Autodesk Inventor part; units mm, degrees
(part 3 of 3)
  line L539 (30.1684, 3.8123) -> (30.5948, 3.6909)
  line L540 (30.5948, 3.6909) -> (31.0222, 3.5524)
  line L541 (31.0222, 3.5524) -> (31.0829, 2.9751)
  line L542 (31.0829, 2.9751) -> (30.6936, 2.7507)
  line L543 (30.6936, 2.7507) -> (30.3018, 2.5433)
  line L544 (30.3018, 2.5433) -> (29.9075, 2.3538)
  line L545 (29.9075, 2.3538) -> (29.511, 2.1835)
  line L546 (29.511, 2.1835) -> (29.1124, 2.0344)
  line L547 (29.1124, 2.0344) -> (28.9123, 1.9688)
  line L548 (28.9123, 1.9688) -> (28.812, 1.9385)
  line L549 (28.812, 1.9385) -> (28.7116, 1.9099)
  line L550 (28.7116, 1.9099) -> (28.754, 1.1017)
  line L551 (28.754, 1.1017) -> (28.8568, 1.0838)
  line L552 (28.8568, 1.0838) -> (28.9597, 1.0641)
  line L553 (28.9597, 1.0641) -> (29.1656, 1.0198)
  line L554 (29.1656, 1.0198) -> (29.5776, 0.9132)
  line L555 (29.5776, 0.9132) -> (29.9897, 0.7853)
  line L556 (29.9897, 0.7853) -> (30.4016, 0.638)
  line L557 (30.4016, 0.638) -> (30.813, 0.4727)
  line L558 (30.813, 0.4727) -> (31.2236, 0.2903)
  line L559 (31.2236, 0.2903) -> (31.2236, -0.2903)
  line L560 (31.2236, -0.2903) -> (30.813, -0.4727)
  line L561 (30.813, -0.4727) -> (30.4016, -0.638)
  line L562 (30.4016, -0.638) -> (29.9897, -0.7853)
  line L563 (29.9897, -0.7853) -> (29.5776, -0.9132)
  line L564 (29.5776, -0.9132) -> (29.1656, -1.0198)
  line L565 (29.1656, -1.0198) -> (28.9597, -1.0641)
  line L566 (28.9597, -1.0641) -> (28.8568, -1.0838)
  line L567 (28.8568, -1.0838) -> (28.754, -1.1017)
  line L568 (28.754, -1.1017) -> (28.7116, -1.9099)
  line L569 (28.7116, -1.9099) -> (28.812, -1.9385)
  line L570 (28.812, -1.9385) -> (28.9123, -1.9688)
  line L571 (28.9123, -1.9688) -> (29.1124, -2.0344)
  line L572 (29.1124, -2.0344) -> (29.511, -2.1835)
  line L573 (29.511, -2.1835) -> (29.9075, -2.3538)
  line L574 (29.9075, -2.3538) -> (30.3018, -2.5433)
  line L575 (30.3018, -2.5433) -> (30.6936, -2.7507)
  line L576 (30.6936, -2.7507) -> (31.0829, -2.9751)
  line L577 (31.0829, -2.9751) -> (31.0222, -3.5524)
  line L578 (31.0222, -3.5524) -> (30.5948, -3.6909)
  line L579 (30.5948, -3.6909) -> (30.1684, -3.8124)
  line L580 (30.1684, -3.8124) -> (29.7433, -3.9158)
  line L581 (29.7433, -3.9158) -> (29.3201, -3.9999)
  line L582 (29.3201, -3.9999) -> (28.8992, -4.0628)
  line L583 (28.8992, -4.0628) -> (28.6898, -4.0854)
  line L584 (28.6898, -4.0854) -> (28.5855, -4.0942)
  line L585 (28.5855, -4.0942) -> (28.4813, -4.1013)
  line L586 (28.4813, -4.1013) -> (28.3547, -4.9006)
  line L587 (28.3547, -4.9006) -> (28.4516, -4.9395)
  line L588 (28.4516, -4.9395) -> (28.5481, -4.9802)
  line L589 (28.5481, -4.9802) -> (28.7403, -5.0663)
  line L590 (28.7403, -5.0663) -> (29.1211, -5.2563)
  line L591 (29.1211, -5.2563) -> (29.4976, -5.4671)
  line L592 (29.4976, -5.4671) -> (29.8699, -5.6968)
  line L593 (29.8699, -5.6968) -> (30.2379, -5.944)
  line L594 (30.2379, -5.944) -> (30.6016, -6.2078)
  line L595 (30.6016, -6.2078) -> (30.4809, -6.7757)
  line L596 (30.4809, -6.7757) -> (30.0414, -6.8687)
  line L597 (30.0414, -6.8687) -> (29.6046, -6.9449)
  line L598 (29.6046, -6.9449) -> (29.1711, -7.0034)
  line L599 (29.1711, -7.0034) -> (28.7414, -7.0428)
  line L600 (28.7414, -7.0428) -> (28.3162, -7.0614)
  line L601 (28.3162, -7.0614) -> (28.1056, -7.0619)
  line L602 (28.1056, -7.0619) -> (28.0009, -7.0598)
  line L603 (28.0009, -7.0598) -> (27.8966, -7.0559)
  line L604 (27.8966, -7.0559) -> (27.6871, -7.8377)
  line L605 (27.6871, -7.8377) -> (27.7794, -7.8865)
  line L606 (27.7794, -7.8865) -> (27.8711, -7.937)
  line L607 (27.8711, -7.937) -> (28.0532, -8.0428)
  line L608 (28.0532, -8.0428) -> (28.4122, -8.2714)
  line L609 (28.4122, -8.2714) -> (28.7646, -8.5205)
  line L610 (28.7646, -8.5205) -> (29.1108, -8.7878)
  line L611 (29.1108, -8.7878) -> (29.451, -9.0722)
  line L612 (29.451, -9.0722) -> (29.7851, -9.3725)
  line L613 (29.7851, -9.3725) -> (29.6057, -9.9247)
  line L614 (29.6057, -9.9247) -> (29.1588, -9.9713)
  line L615 (29.1588, -9.9713) -> (28.7165, -10.0014)
  line L616 (28.7165, -10.0014) -> (28.2792, -10.0142)
  line L617 (28.2792, -10.0142) -> (27.8478, -10.0085)
  line L618 (27.8478, -10.0085) -> (27.423, -9.9825)
  line L619 (27.423, -9.9825) -> (27.2135, -9.9611)
  line L620 (27.2135, -9.9611) -> (27.1095, -9.948)
  line L621 (27.1095, -9.948) -> (27.0062, -9.9333)
  line L622 (27.0062, -9.9333) -> (26.7162, -10.6888)
  line L623 (26.7162, -10.6888) -> (26.8028, -10.747)
  line L624 (26.8028, -10.747) -> (26.8888, -10.8068)
  line L625 (26.8888, -10.8068) -> (27.0589, -10.9311)
  line L626 (27.0589, -10.9311) -> (27.3919, -11.196)
  line L627 (27.3919, -11.196) -> (27.7164, -11.4805)
  line L628 (27.7164, -11.4805) -> (28.0328, -11.7826)
  line L629 (28.0328, -11.7826) -> (28.3413, -12.1009)
  line L630 (28.3413, -12.1009) -> (28.6422, -12.4346)
  line L631 (28.6422, -12.4346) -> (28.4061, -12.965)
  line L632 (28.4061, -12.965) -> (27.9568, -12.9646)
  line L633 (27.9568, -12.9646) -> (27.5137, -12.9483)
  line L634 (27.5137, -12.9483) -> (27.0776, -12.9153)
  line L635 (27.0776, -12.9153) -> (26.649, -12.8646)
  line L636 (26.649, -12.8646) -> (26.2293, -12.7943)
  line L637 (26.2293, -12.7943) -> (26.0232, -12.7511)
  line L638 (26.0232, -12.7511) -> (25.9212, -12.7272)
  line L639 (25.9212, -12.7272) -> (25.82, -12.7018)
  line L640 (25.82, -12.7018) -> (25.4526, -13.4229)
  line L641 (25.4526, -13.4229) -> (25.5327, -13.4898)
  line L642 (25.5327, -13.4898) -> (25.6119, -13.5583)
  line L643 (25.6119, -13.5583) -> (25.768, -13.6996)
  line L644 (25.768, -13.6996) -> (26.0716, -13.9979)
  line L645 (26.0716, -13.9979) -> (26.3645, -14.3148)
  line L646 (26.3645, -14.3148) -> (26.6476, -14.6483)
  line L647 (26.6476, -14.6483) -> (26.9212, -14.9971)
  line L648 (26.9212, -14.9971) -> (27.1855, -15.3604)
  line L649 (27.1855, -15.3604) -> (26.8952, -15.8632)
  line L650 (26.8952, -15.8632) -> (26.4485, -15.8158)
  line L651 (26.4485, -15.8158) -> (26.0096, -15.7533)
  line L652 (26.0096, -15.7533) -> (25.5792, -15.675)
  line L653 (25.5792, -15.675) -> (25.1583, -15.5797)
  line L654 (25.1583, -15.5797) -> (24.7482, -15.466)
  line L655 (24.7482, -15.466) -> (24.5478, -15.4014)
  line L656 (24.5478, -15.4014) -> (24.4488, -15.367)
  line L657 (24.4488, -15.367) -> (24.3508, -15.3311)
  line L658 (24.3508, -15.3311) -> (23.91, -16.0099)
  line L659 (23.91, -16.0099) -> (23.9827, -16.0848)
  line L660 (23.9827, -16.0848) -> (24.0544, -16.1612)
  line L661 (24.0544, -16.1612) -> (24.1949, -16.3181)
  line L662 (24.1949, -16.3181) -> (24.4656, -16.6465)
  line L663 (24.4656, -16.6465) -> (24.7238, -16.9922)
  line L664 (24.7238, -16.9922) -> (24.9704, -17.3534)
  line L665 (24.9704, -17.3534) -> (25.2061, -17.729)
  line L666 (25.2061, -17.729) -> (25.431, -18.1179)
  line L667 (25.431, -18.1179) -> (25.0898, -18.5876)
  line L668 (25.0898, -18.5876) -> (24.6504, -18.4938)
  line L669 (24.6504, -18.4938) -> (24.2204, -18.3858)
  line L670 (24.2204, -18.3858) -> (23.8006, -18.2628)
  line L671 (23.8006, -18.2628) -> (23.392, -18.1241)
  line L672 (23.392, -18.1241) -> (22.996, -17.9681)
  line L673 (22.996, -17.9681) -> (22.8034, -17.883)
  line L674 (22.8034, -17.883) -> (22.7086, -17.8384)
  line L675 (22.7086, -17.8384) -> (22.6149, -17.7925)
  line L676 (22.6149, -17.7925) -> (22.1056, -18.4214)
  line L677 (22.1056, -18.4214) -> (22.17, -18.5035)
  line L678 (22.17, -18.5035) -> (22.2333, -18.587)
  line L679 (22.2333, -18.587) -> (22.3566, -18.7577)
  line L680 (22.3566, -18.7577) -> (22.5915, -19.1126)
  line L681 (22.5915, -19.1126) -> (22.8122, -19.4834)
  line L682 (22.8122, -19.4834) -> (23.0197, -19.8685)
  line L683 (23.0197, -19.8685) -> (23.2148, -20.2666)
  line L684 (23.2148, -20.2666) -> (23.3979, -20.6769)
  line L685 (23.3979, -20.6769) -> (23.0094, -21.1084)
  line L686 (23.0094, -21.1084) -> (22.5822, -20.9692)
  line L687 (22.5822, -20.9692) -> (22.1659, -20.8168)
  line L688 (22.1659, -20.8168) -> (21.7612, -20.6506)
  line L689 (21.7612, -20.6506) -> (21.3694, -20.4699)
  line L690 (21.3694, -20.4699) -> (20.9919, -20.2734)
  line L691 (20.9919, -20.2734) -> (20.8092, -20.1686)
  line L692 (20.8092, -20.1686) -> (20.7196, -20.1144)
  line L693 (20.7196, -20.1144) -> (20.6312, -20.0589)
  line L694 (20.6312, -20.0589) -> (20.0589, -20.6312)
  line L695 (20.0589, -20.6312) -> (20.1144, -20.7196)
  line L696 (20.1144, -20.7196) -> (20.1686, -20.8092)
  line L697 (20.1686, -20.8092) -> (20.2734, -20.9919)
  line L698 (20.2734, -20.9919) -> (20.4699, -21.3694)
  line L699 (20.4699, -21.3694) -> (20.6506, -21.7612)
  line L700 (20.6506, -21.7612) -> (20.8168, -22.1659)
  line L701 (20.8168, -22.1659) -> (20.9692, -22.5822)
  line L702 (20.9692, -22.5822) -> (21.1084, -23.0094)
  line L703 (21.1084, -23.0094) -> (20.6769, -23.3979)
  line L704 (20.6769, -23.3979) -> (20.2666, -23.2148)
  line L705 (20.2666, -23.2148) -> (19.8685, -23.0197)
  line L706 (19.8685, -23.0197) -> (19.4834, -22.8122)
  line L707 (19.4834, -22.8122) -> (19.1126, -22.5915)
  line L708 (19.1126, -22.5915) -> (18.7577, -22.3566)
  line L709 (18.7577, -22.3566) -> (18.587, -22.2333)
  line L710 (18.587, -22.2333) -> (18.5035, -22.17)
  line L711 (18.5035, -22.17) -> (18.4214, -22.1056)
  line L712 (18.4214, -22.1056) -> (17.7925, -22.6149)
  line L713 (17.7925, -22.6149) -> (17.8384, -22.7086)
  line L714 (17.8384, -22.7086) -> (17.883, -22.8034)
  line L715 (17.883, -22.8034) -> (17.9681, -22.996)
  line L716 (17.9681, -22.996) -> (18.1241, -23.392)
  line L717 (18.1241, -23.392) -> (18.2628, -23.8006)
  line L718 (18.2628, -23.8006) -> (18.3858, -24.2204)
  line L719 (18.3858, -24.2204) -> (18.4938, -24.6504)
  line L720 (18.4938, -24.6504) -> (18.5876, -25.0898)
  line L721 (18.5876, -25.0898) -> (18.1179, -25.431)
  line L722 (18.1179, -25.431) -> (17.729, -25.2061)
  line L723 (17.729, -25.2061) -> (17.3535, -24.9704)
  line L724 (17.3535, -24.9704) -> (16.9922, -24.7238)
  line L725 (16.9922, -24.7238) -> (16.6465, -24.4656)
  line L726 (16.6465, -24.4656) -> (16.3181, -24.1949)
  line L727 (16.3181, -24.1949) -> (16.1612, -24.0544)
  line L728 (16.1612, -24.0544) -> (16.0848, -23.9827)
  line L729 (16.0848, -23.9827) -> (16.0099, -23.91)
  line L730 (16.0099, -23.91) -> (15.3311, -24.3508)
  line L731 (15.3311, -24.3508) -> (15.367, -24.4488)
  line L732 (15.367, -24.4488) -> (15.4014, -24.5478)
  line L733 (15.4014, -24.5478) -> (15.466, -24.7482)
  line L734 (15.466, -24.7482) -> (15.5797, -25.1583)
  line L735 (15.5797, -25.1583) -> (15.675, -25.5792)
  line L736 (15.675, -25.5792) -> (15.7533, -26.0096)
  line L737 (15.7533, -26.0096) -> (15.8158, -26.4485)
  line L738 (15.8158, -26.4485) -> (15.8632, -26.8952)
  line L739 (15.8632, -26.8952) -> (15.3604, -27.1855)
  line L740 (15.3604, -27.1855) -> (14.9971, -26.9212)
  line L741 (14.9971, -26.9212) -> (14.6483, -26.6476)
  line L742 (14.6483, -26.6476) -> (14.3148, -26.3645)
  line L743 (14.3148, -26.3645) -> (13.9979, -26.0716)
  line L744 (13.9979, -26.0716) -> (13.6996, -25.768)
  line L745 (13.6996, -25.768) -> (13.5583, -25.6119)
  line L746 (13.5583, -25.6119) -> (13.4898, -25.5326)
  line L747 (13.4898, -25.5326) -> (13.4229, -25.4525)
  line L748 (13.4229, -25.4525) -> (12.7018, -25.82)
  line L749 (12.7018, -25.82) -> (12.7272, -25.9212)
  line L750 (12.7272, -25.9212) -> (12.7511, -26.0232)
  line L751 (12.7511, -26.0232) -> (12.7943, -26.2293)
  line L752 (12.7943, -26.2293) -> (12.8646, -26.649)
  line L753 (12.8646, -26.649) -> (12.9153, -27.0776)
  line L754 (12.9153, -27.0776) -> (12.9483, -27.5137)
  line L755 (12.9483, -27.5137) -> (12.9646, -27.9568)
  line L756 (12.9646, -27.9568) -> (12.965, -28.4061)
  line L757 (12.965, -28.4061) -> (12.4346, -28.6422)
  line L758 (12.4346, -28.6422) -> (12.1009, -28.3413)
  line L759 (12.1009, -28.3413) -> (11.7826, -28.0328)
  line L760 (11.7826, -28.0328) -> (11.4805, -27.7164)
  line L761 (11.4805, -27.7164) -> (11.196, -27.3919)
  line L762 (11.196, -27.3919) -> (10.9311, -27.0589)
  line L763 (10.9311, -27.0589) -> (10.8068, -26.8888)
  line L764 (10.8068, -26.8888) -> (10.747, -26.8029)
  line L765 (10.747, -26.8029) -> (10.6888, -26.7162)
  line L766 (10.6888, -26.7162) -> (9.9333, -27.0062)
  line L767 (9.9333, -27.0062) -> (9.948, -27.1095)
  line L768 (9.948, -27.1095) -> (9.9611, -27.2135)
  line L769 (9.9611, -27.2135) -> (9.9825, -27.423)
  line L770 (9.9825, -27.423) -> (10.0085, -27.8478)
  line L771 (10.0085, -27.8478) -> (10.0142, -28.2792)
  line L772 (10.0142, -28.2792) -> (10.0014, -28.7165)
  line L773 (10.0014, -28.7165) -> (9.9713, -29.1588)
  line L774 (9.9713, -29.1588) -> (9.9247, -29.6057)
  line L775 (9.9247, -29.6057) -> (9.3725, -29.7851)
  line L776 (9.3725, -29.7851) -> (9.0722, -29.4509)
  line L777 (9.0722, -29.4509) -> (8.7878, -29.1108)
  line L778 (8.7878, -29.1108) -> (8.5205, -28.7646)
  line L779 (8.5205, -28.7646) -> (8.2714, -28.4122)
  line L780 (8.2714, -28.4122) -> (8.0428, -28.0532)
  line L781 (8.0428, -28.0532) -> (7.937, -27.8711)
  line L782 (7.937, -27.8711) -> (7.8865, -27.7794)
  line L783 (7.8865, -27.7794) -> (7.8377, -27.6871)
  line L784 (7.8377, -27.6871) -> (7.0559, -27.8966)
  line L785 (7.0559, -27.8966) -> (7.0598, -28.0009)
  line L786 (7.0598, -28.0009) -> (7.0619, -28.1056)
  line L787 (7.0619, -28.1056) -> (7.0614, -28.3162)
  line L788 (7.0614, -28.3162) -> (7.0428, -28.7414)
  line L789 (7.0428, -28.7414) -> (7.0034, -29.1711)
  line L790 (7.0034, -29.1711) -> (6.9449, -29.6046)
  line L791 (6.9449, -29.6046) -> (6.8687, -30.0414)
  line L792 (6.8687, -30.0414) -> (6.7757, -30.4809)
  line L793 (6.7757, -30.4809) -> (6.2078, -30.6016)
  line L794 (6.2078, -30.6016) -> (5.944, -30.2379)
  line L795 (5.944, -30.2379) -> (5.6968, -29.8699)
  line L796 (5.6968, -29.8699) -> (5.4671, -29.4976)
  line L797 (5.4671, -29.4976) -> (5.2563, -29.1211)
  line L798 (5.2563, -29.1211) -> (5.0664, -28.7403)
  line L799 (5.0664, -28.7403) -> (4.9802, -28.5481)
  line L800 (4.9802, -28.5481) -> (4.9395, -28.4516)
  line L801 (4.9395, -28.4516) -> (4.9006, -28.3547)
  line L802 (4.9006, -28.3547) -> (4.1013, -28.4813)
  line L803 (4.1013, -28.4813) -> (4.0942, -28.5854)
  line L804 (4.0942, -28.5854) -> (4.0854, -28.6898)
  line L805 (4.0854, -28.6898) -> (4.0628, -28.8992)
  line L806 (4.0628, -28.8992) -> (3.9999, -29.3201)
  line L807 (3.9999, -29.3201) -> (3.9158, -29.7433)
  line L808 (3.9158, -29.7433) -> (3.8123, -30.1684)
  line L809 (3.8123, -30.1684) -> (3.6909, -30.5948)
  line L810 (3.6909, -30.5948) -> (3.5524, -31.0222)
  line L811 (3.5524, -31.0222) -> (2.975, -31.0829)
  line L812 (2.975, -31.0829) -> (2.7507, -30.6936)
  line L813 (2.7507, -30.6936) -> (2.5433, -30.3017)
  line L814 (2.5433, -30.3017) -> (2.3538, -29.9075)
  line L815 (2.3538, -29.9075) -> (2.1835, -29.511)
  line L816 (2.1835, -29.511) -> (2.0344, -29.1124)
  line L817 (2.0344, -29.1124) -> (1.9688, -28.9123)
  line L818 (1.9688, -28.9123) -> (1.9385, -28.812)
  line L819 (1.9385, -28.812) -> (1.9099, -28.7116)
  line L820 (1.9099, -28.7116) -> (1.1017, -28.754)
  line L821 (1.1017, -28.754) -> (1.0838, -28.8568)
  line L822 (1.0838, -28.8568) -> (1.0641, -28.9597)
  line L823 (1.0641, -28.9597) -> (1.0198, -29.1656)
  line L824 (1.0198, -29.1656) -> (0.9132, -29.5776)
  line L825 (0.9132, -29.5776) -> (0.7853, -29.9897)
  line L826 (0.7853, -29.9897) -> (0.638, -30.4016)
  line L827 (0.638, -30.4016) -> (0.4727, -30.813)
  line L828 (0.4727, -30.813) -> (0.2903, -31.2236)
  line L829 (0.2903, -31.2236) -> (-0.2903, -31.2236)
  line L830 (-0.2903, -31.2236) -> (-0.4727, -30.813)
  line L831 (-0.4727, -30.813) -> (-0.638, -30.4016)
  line L832 (-0.638, -30.4016) -> (-0.7853, -29.9897)
  line L833 (-0.7853, -29.9897) -> (-0.9132, -29.5776)
  line L834 (-0.9132, -29.5776) -> (-1.0198, -29.1656)
  line L835 (-1.0198, -29.1656) -> (-1.0641, -28.9597)
  line L836 (-1.0641, -28.9597) -> (-1.0838, -28.8568)
  line L837 (-1.0838, -28.8568) -> (-1.1017, -28.754)
  line L838 (-1.1017, -28.754) -> (-1.9099, -28.7116)
  line L839 (-1.9099, -28.7116) -> (-1.9385, -28.812)
  line L840 (-1.9385, -28.812) -> (-1.9688, -28.9123)
  line L841 (-1.9688, -28.9123) -> (-2.0344, -29.1124)
  line L842 (-2.0344, -29.1124) -> (-2.1835, -29.511)
  line L843 (-2.1835, -29.511) -> (-2.3538, -29.9075)
  line L844 (-2.3538, -29.9075) -> (-2.5433, -30.3018)
  line L845 (-2.5433, -30.3018) -> (-2.7507, -30.6936)
  line L846 (-2.7507, -30.6936) -> (-2.9751, -31.0829)
  line L847 (-2.9751, -31.0829) -> (-3.5525, -31.0222)
  line L848 (-3.5525, -31.0222) -> (-3.6909, -30.5948)
  line L849 (-3.6909, -30.5948) -> (-3.8124, -30.1684)
  line L850 (-3.8124, -30.1684) -> (-3.9158, -29.7433)
  line L851 (-3.9158, -29.7433) -> (-3.9999, -29.3201)
  line L852 (-3.9999, -29.3201) -> (-4.0628, -28.8992)
  line L853 (-4.0628, -28.8992) -> (-4.0854, -28.6898)
  line L854 (-4.0854, -28.6898) -> (-4.0942, -28.5855)
  line L855 (-4.0942, -28.5855) -> (-4.1013, -28.4813)
  line L856 (-4.1013, -28.4813) -> (-4.9006, -28.3547)
  line L857 (-4.9006, -28.3547) -> (-4.9395, -28.4516)
  line L858 (-4.9395, -28.4516) -> (-4.9802, -28.5481)
  line L859 (-4.9802, -28.5481) -> (-5.0663, -28.7403)
  line L860 (-5.0663, -28.7403) -> (-5.2563, -29.1211)
  line L861 (-5.2563, -29.1211) -> (-5.4671, -29.4976)
  line L862 (-5.4671, -29.4976) -> (-5.6968, -29.8699)
  line L863 (-5.6968, -29.8699) -> (-5.944, -30.2379)
  line L864 (-5.944, -30.2379) -> (-6.2078, -30.6016)
  line L865 (-6.2078, -30.6016) -> (-6.7757, -30.4809)
  line L866 (-6.7757, -30.4809) -> (-6.8687, -30.0414)
  line L867 (-6.8687, -30.0414) -> (-6.9449, -29.6046)
  line L868 (-6.9449, -29.6046) -> (-7.0034, -29.1711)
  line L869 (-7.0034, -29.1711) -> (-7.0428, -28.7414)
  line L870 (-7.0428, -28.7414) -> (-7.0614, -28.3162)
  line L871 (-7.0614, -28.3162) -> (-7.0619, -28.1056)
  line L872 (-7.0619, -28.1056) -> (-7.0598, -28.0009)
  line L873 (-7.0598, -28.0009) -> (-7.0559, -27.8966)
  line L874 (-7.0559, -27.8966) -> (-7.8377, -27.6871)
  line L875 (-7.8377, -27.6871) -> (-7.8865, -27.7794)
  line L876 (-7.8865, -27.7794) -> (-7.937, -27.8711)
  line L877 (-7.937, -27.8711) -> (-8.0428, -28.0532)
  line L878 (-8.0428, -28.0532) -> (-8.2715, -28.4122)
  line L879 (-8.2715, -28.4122) -> (-8.5205, -28.7646)
  line L880 (-8.5205, -28.7646) -> (-8.7878, -29.1108)
  line L881 (-8.7878, -29.1108) -> (-9.0722, -29.4509)
  line L882 (-9.0722, -29.4509) -> (-9.3725, -29.7851)
  line L883 (-9.3725, -29.7851) -> (-9.9247, -29.6057)
  line L884 (-9.9247, -29.6057) -> (-9.9713, -29.1588)
  line L885 (-9.9713, -29.1588) -> (-10.0014, -28.7165)
  line L886 (-10.0014, -28.7165) -> (-10.0142, -28.2792)
  line L887 (-10.0142, -28.2792) -> (-10.0085, -27.8478)
  line L888 (-10.0085, -27.8478) -> (-9.9825, -27.423)
  line L889 (-9.9825, -27.423) -> (-9.9611, -27.2135)
  line L890 (-9.9611, -27.2135) -> (-9.948, -27.1095)
  line L891 (-9.948, -27.1095) -> (-9.9333, -27.0062)
  line L892 (-9.9333, -27.0062) -> (-10.6888, -26.7162)
  line L893 (-10.6888, -26.7162) -> (-10.747, -26.8028)
  line L894 (-10.747, -26.8028) -> (-10.8068, -26.8888)
  line L895 (-10.8068, -26.8888) -> (-10.9311, -27.0589)
  line L896 (-10.9311, -27.0589) -> (-11.196, -27.3919)
  line L897 (-11.196, -27.3919) -> (-11.4805, -27.7164)
  line L898 (-11.4805, -27.7164) -> (-11.7826, -28.0327)
  line L899 (-11.7826, -28.0327) -> (-12.101, -28.3413)
  line L900 (-12.101, -28.3413) -> (-12.4346, -28.6422)
  line L901 (-12.4346, -28.6422) -> (-12.965, -28.4061)
  line L902 (-12.965, -28.4061) -> (-12.9646, -27.9568)
  line L903 (-12.9646, -27.9568) -> (-12.9483, -27.5137)
  line L904 (-12.9483, -27.5137) -> (-12.9153, -27.0776)
  line L905 (-12.9153, -27.0776) -> (-12.8646, -26.649)
  line L906 (-12.8646, -26.649) -> (-12.7943, -26.2293)
  line L907 (-12.7943, -26.2293) -> (-12.7511, -26.0232)
  line L908 (-12.7511, -26.0232) -> (-12.7273, -25.9212)
  line L909 (-12.7273, -25.9212) -> (-12.7018, -25.82)
  line L910 (-12.7018, -25.82) -> (-13.4229, -25.4525)
  line L911 (-13.4229, -25.4525) -> (-13.4898, -25.5327)
  line L912 (-13.4898, -25.5327) -> (-13.5583, -25.6119)
  line L913 (-13.5583, -25.6119) -> (-13.6996, -25.768)
  line L914 (-13.6996, -25.768) -> (-13.9979, -26.0716)
  line L915 (-13.9979, -26.0716) -> (-14.3148, -26.3645)
  line L916 (-14.3148, -26.3645) -> (-14.6483, -26.6476)
  line L917 (-14.6483, -26.6476) -> (-14.9971, -26.9212)
  line L918 (-14.9971, -26.9212) -> (-15.3604, -27.1855)
  line L919 (-15.3604, -27.1855) -> (-15.8632, -26.8952)
  line L920 (-15.8632, -26.8952) -> (-15.8158, -26.4485)
  line L921 (-15.8158, -26.4485) -> (-15.7533, -26.0096)
  line L922 (-15.7533, -26.0096) -> (-15.675, -25.5792)
  line L923 (-15.675, -25.5792) -> (-15.5797, -25.1583)
  line L924 (-15.5797, -25.1583) -> (-15.466, -24.7482)
  line L925 (-15.466, -24.7482) -> (-15.4014, -24.5478)
  line L926 (-15.4014, -24.5478) -> (-15.367, -24.4488)
  line L927 (-15.367, -24.4488) -> (-15.3311, -24.3508)
  line L928 (-15.3311, -24.3508) -> (-16.0099, -23.91)
  line L929 (-16.0099, -23.91) -> (-16.0848, -23.9827)
  line L930 (-16.0848, -23.9827) -> (-16.1612, -24.0544)
  line L931 (-16.1612, -24.0544) -> (-16.3181, -24.1949)
  line L932 (-16.3181, -24.1949) -> (-16.6465, -24.4656)
  line L933 (-16.6465, -24.4656) -> (-16.9922, -24.7238)
  line L934 (-16.9922, -24.7238) -> (-17.3535, -24.9704)
  line L935 (-17.3535, -24.9704) -> (-17.729, -25.2061)
  line L936 (-17.729, -25.2061) -> (-18.1179, -25.431)
  line L937 (-18.1179, -25.431) -> (-18.5876, -25.0898)
  line L938 (-18.5876, -25.0898) -> (-18.4938, -24.6504)
  line L939 (-18.4938, -24.6504) -> (-18.3858, -24.2204)
  line L940 (-18.3858, -24.2204) -> (-18.2628, -23.8006)
  line L941 (-18.2628, -23.8006) -> (-18.1241, -23.392)
  line L942 (-18.1241, -23.392) -> (-17.9681, -22.996)
  line L943 (-17.9681, -22.996) -> (-17.883, -22.8034)
  line L944 (-17.883, -22.8034) -> (-17.8384, -22.7086)
  line L945 (-17.8384, -22.7086) -> (-17.7925, -22.6149)
  line L946 (-17.7925, -22.6149) -> (-18.4214, -22.1056)
  line L947 (-18.4214, -22.1056) -> (-18.5035, -22.17)
  line L948 (-18.5035, -22.17) -> (-18.587, -22.2333)
  line L949 (-18.587, -22.2333) -> (-18.7577, -22.3566)
  line L950 (-18.7577, -22.3566) -> (-19.1126, -22.5915)
  line L951 (-19.1126, -22.5915) -> (-19.4834, -22.8122)
  line L952 (-19.4834, -22.8122) -> (-19.8685, -23.0197)
  line L953 (-19.8685, -23.0197) -> (-20.2666, -23.2148)
  line L954 (-20.2666, -23.2148) -> (-20.6769, -23.3979)
  line L955 (-20.6769, -23.3979) -> (-21.1084, -23.0094)
  line L956 (-21.1084, -23.0094) -> (-20.9692, -22.5822)
  line L957 (-20.9692, -22.5822) -> (-20.8168, -22.1659)
  line L958 (-20.8168, -22.1659) -> (-20.6506, -21.7612)
  line L959 (-20.6506, -21.7612) -> (-20.4699, -21.3694)
  line L960 (-20.4699, -21.3694) -> (-20.2734, -20.9919)
  line L961 (-20.2734, -20.9919) -> (-20.1686, -20.8092)
  line L962 (-20.1686, -20.8092) -> (-20.1144, -20.7196)
  line L963 (-20.1144, -20.7196) -> (-20.0589, -20.6312)
  line L964 (-20.0589, -20.6312) -> (-20.6312, -20.0589)
  line L965 (-20.6312, -20.0589) -> (-20.7196, -20.1144)
  line L966 (-20.7196, -20.1144) -> (-20.8092, -20.1686)
  line L967 (-20.8092, -20.1686) -> (-20.9919, -20.2734)
  line L968 (-20.9919, -20.2734) -> (-21.3694, -20.4699)
  line L969 (-21.3694, -20.4699) -> (-21.7612, -20.6506)
  line L970 (-21.7612, -20.6506) -> (-22.1659, -20.8168)
  line L971 (-22.1659, -20.8168) -> (-22.5822, -20.9692)
  line L972 (-22.5822, -20.9692) -> (-23.0094, -21.1084)
  line L973 (-23.0094, -21.1084) -> (-23.3979, -20.6769)
  line L974 (-23.3979, -20.6769) -> (-23.2148, -20.2666)
  line L975 (-23.2148, -20.2666) -> (-23.0197, -19.8685)
  line L976 (-23.0197, -19.8685) -> (-22.8122, -19.4834)
  line L977 (-22.8122, -19.4834) -> (-22.5915, -19.1126)
  line L978 (-22.5915, -19.1126) -> (-22.3566, -18.7577)
  line L979 (-22.3566, -18.7577) -> (-22.2333, -18.587)
  line L980 (-22.2333, -18.587) -> (-22.17, -18.5035)
  line L981 (-22.17, -18.5035) -> (-22.1056, -18.4214)
  line L982 (-22.1056, -18.4214) -> (-22.6149, -17.7925)
  line L983 (-22.6149, -17.7925) -> (-22.7086, -17.8384)
  line L984 (-22.7086, -17.8384) -> (-22.8034, -17.883)
  line L985 (-22.8034, -17.883) -> (-22.996, -17.9681)
  line L986 (-22.996, -17.9681) -> (-23.392, -18.1241)
  line L987 (-23.392, -18.1241) -> (-23.8006, -18.2628)
  line L988 (-23.8006, -18.2628) -> (-24.2204, -18.3858)
  line L989 (-24.2204, -18.3858) -> (-24.6504, -18.4938)
  line L990 (-24.6504, -18.4938) -> (-25.0898, -18.5876)
  line L991 (-25.0898, -18.5876) -> (-25.431, -18.1179)
  line L992 (-25.431, -18.1179) -> (-25.2061, -17.729)
  line L993 (-25.2061, -17.729) -> (-24.9704, -17.3535)
  line L994 (-24.9704, -17.3535) -> (-24.7238, -16.9922)
  line L995 (-24.7238, -16.9922) -> (-24.4656, -16.6465)
  line L996 (-24.4656, -16.6465) -> (-24.1949, -16.3181)
  line L997 (-24.1949, -16.3181) -> (-24.0544, -16.1612)
  line L998 (-24.0544, -16.1612) -> (-23.9827, -16.0848)
  line L999 (-23.9827, -16.0848) -> (-23.91, -16.0099)
  line L1000 (-23.91, -16.0099) -> (-24.3508, -15.3311)
  line L1001 (-24.3508, -15.3311) -> (-24.4488, -15.367)
  line L1002 (-24.4488, -15.367) -> (-24.5478, -15.4014)
  line L1003 (-24.5478, -15.4014) -> (-24.7482, -15.4659)
  line L1004 (-24.7482, -15.4659) -> (-25.1583, -15.5797)
  line L1005 (-25.1583, -15.5797) -> (-25.5792, -15.675)
  line L1006 (-25.5792, -15.675) -> (-26.0096, -15.7533)
  line L1007 (-26.0096, -15.7533) -> (-26.4485, -15.8158)
  line L1008 (-26.4485, -15.8158) -> (-26.8953, -15.8632)
  line L1009 (-26.8953, -15.8632) -> (-27.1855, -15.3604)
  line L1010 (-27.1855, -15.3604) -> (-26.9212, -14.9971)
  line L1011 (-26.9212, -14.9971) -> (-26.6476, -14.6483)
  line L1012 (-26.6476, -14.6483) -> (-26.3645, -14.3148)
  line L1013 (-26.3645, -14.3148) -> (-26.0716, -13.9979)
  line L1014 (-26.0716, -13.9979) -> (-25.768, -13.6996)
  line L1015 (-25.768, -13.6996) -> (-25.6119, -13.5583)
  line L1016 (-25.6119, -13.5583) -> (-25.5327, -13.4898)
  line L1017 (-25.5327, -13.4898) -> (-25.4525, -13.4229)
  line L1018 (-25.4525, -13.4229) -> (-25.82, -12.7018)
  line L1019 (-25.82, -12.7018) -> (-25.9212, -12.7272)
  line L1020 (-25.9212, -12.7272) -> (-26.0232, -12.7511)
  line L1021 (-26.0232, -12.7511) -> (-26.2293, -12.7943)
  line L1022 (-26.2293, -12.7943) -> (-26.649, -12.8646)
  line L1023 (-26.649, -12.8646) -> (-27.0776, -12.9153)
  line L1024 (-27.0776, -12.9153) -> (-27.5137, -12.9483)
  line L1025 (-27.5137, -12.9483) -> (-27.9568, -12.9646)
  line L1026 (-27.9568, -12.9646) -> (-28.4061, -12.965)
  line L1027 (-28.4061, -12.965) -> (-28.6422, -12.4346)
  line L1028 (-28.6422, -12.4346) -> (-28.3413, -12.1009)
  line L1029 (-28.3413, -12.1009) -> (-28.0328, -11.7826)
  line L1030 (-28.0328, -11.7826) -> (-27.7164, -11.4805)
  line L1031 (-27.7164, -11.4805) -> (-27.3919, -11.196)
  line L1032 (-27.3919, -11.196) -> (-27.0589, -10.9311)
  line L1033 (-27.0589, -10.9311) -> (-26.8888, -10.8068)
  line L1034 (-26.8888, -10.8068) -> (-26.8029, -10.747)
  line L1035 (-26.8029, -10.747) -> (-26.7162, -10.6888)
  line L1036 (-26.7162, -10.6888) -> (-27.0062, -9.9333)
  line L1037 (-27.0062, -9.9333) -> (-27.1095, -9.948)
  line L1038 (-27.1095, -9.948) -> (-27.2135, -9.9611)
  line L1039 (-27.2135, -9.9611) -> (-27.423, -9.9825)
  line L1040 (-27.423, -9.9825) -> (-27.8478, -10.0085)
  line L1041 (-27.8478, -10.0085) -> (-28.2792, -10.0142)
  line L1042 (-28.2792, -10.0142) -> (-28.7165, -10.0014)
  line L1043 (-28.7165, -10.0014) -> (-29.1588, -9.9713)
  line L1044 (-29.1588, -9.9713) -> (-29.6057, -9.9247)
  line L1045 (-29.6057, -9.9247) -> (-29.7851, -9.3725)
  line L1046 (-29.7851, -9.3725) -> (-29.451, -9.0722)
  line L1047 (-29.451, -9.0722) -> (-29.1108, -8.7878)
  line L1048 (-29.1108, -8.7878) -> (-28.7646, -8.5205)
  line L1049 (-28.7646, -8.5205) -> (-28.4122, -8.2715)
  line L1050 (-28.4122, -8.2715) -> (-28.0532, -8.0428)
  line L1051 (-28.0532, -8.0428) -> (-27.8711, -7.937)
  line L1052 (-27.8711, -7.937) -> (-27.7794, -7.8865)
  line L1053 (-27.7794, -7.8865) -> (-27.6871, -7.8377)
  line L1054 (-27.6871, -7.8377) -> (-27.8966, -7.0559)
  line L1055 (-27.8966, -7.0559) -> (-28.0009, -7.0598)
  line L1056 (-28.0009, -7.0598) -> (-28.1056, -7.0619)
  line L1057 (-28.1056, -7.0619) -> (-28.3162, -7.0614)
  line L1058 (-28.3162, -7.0614) -> (-28.7414, -7.0428)
  line L1059 (-28.7414, -7.0428) -> (-29.1711, -7.0034)
  line L1060 (-29.1711, -7.0034) -> (-29.6046, -6.9449)
  line L1061 (-29.6046, -6.9449) -> (-30.0414, -6.8687)
  line L1062 (-30.0414, -6.8687) -> (-30.4809, -6.7757)
  line L1063 (-30.4809, -6.7757) -> (-30.6016, -6.2078)
  line L1064 (-30.6016, -6.2078) -> (-30.2379, -5.944)
  line L1065 (-30.2379, -5.944) -> (-29.8699, -5.6968)
  line L1066 (-29.8699, -5.6968) -> (-29.4976, -5.4671)
  line L1067 (-29.4976, -5.4671) -> (-29.1211, -5.2563)
  line L1068 (-29.1211, -5.2563) -> (-28.7403, -5.0663)
  line L1069 (-28.7403, -5.0663) -> (-28.5481, -4.9802)
  line L1070 (-28.5481, -4.9802) -> (-28.4516, -4.9395)
  line L1071 (-28.4516, -4.9395) -> (-28.3547, -4.9006)
  line L1072 (-28.3547, -4.9006) -> (-28.4813, -4.1013)
  line L1073 (-28.4813, -4.1013) -> (-28.5854, -4.0942)
  line L1074 (-28.5854, -4.0942) -> (-28.6898, -4.0854)
  line L1075 (-28.6898, -4.0854) -> (-28.8992, -4.0628)
  line L1076 (-28.8992, -4.0628) -> (-29.3201, -3.9999)
  line L1077 (-29.3201, -3.9999) -> (-29.7433, -3.9158)
  line L1078 (-29.7433, -3.9158) -> (-30.1684, -3.8123)
  line L1079 (-30.1684, -3.8123) -> (-30.5948, -3.6909)
  line L1080 (-30.5948, -3.6909) -> (-31.0222, -3.5524)
  line L1081 (-31.0222, -3.5524) -> (-31.0829, -2.9751)
  line L1082 (-31.0829, -2.9751) -> (-30.6936, -2.7507)
  line L1083 (-30.6936, -2.7507) -> (-30.3018, -2.5433)
  line L1084 (-30.3018, -2.5433) -> (-29.9075, -2.3538)
  line L1085 (-29.9075, -2.3538) -> (-29.511, -2.1835)
  line L1086 (-29.511, -2.1835) -> (-29.1124, -2.0344)
  line L1087 (-29.1124, -2.0344) -> (-28.9123, -1.9688)
  line L1088 (-28.9123, -1.9688) -> (-28.812, -1.9385)
  line L1089 (-28.812, -1.9385) -> (-28.7116, -1.9099)
  line L1090 (-28.7116, -1.9099) -> (-28.754, -1.1017)
  line L1091 (-28.754, -1.1017) -> (-28.8568, -1.0838)
  line L1092 (-28.8568, -1.0838) -> (-28.9597, -1.0641)
  line L1093 (-28.9597, -1.0641) -> (-29.1656, -1.0198)
  line L1094 (-29.1656, -1.0198) -> (-29.5776, -0.9132)
  line L1095 (-29.5776, -0.9132) -> (-29.9897, -0.7853)
  line L1096 (-29.9897, -0.7853) -> (-30.4016, -0.638)
  line L1097 (-30.4016, -0.638) -> (-30.813, -0.4727)
  line L1098 (-30.813, -0.4727) -> (-31.2236, -0.2903)
  line L1099 (-31.2236, -0.2903) -> (-31.2236, 0.2903)
  line L1100 (-31.2236, 0.2903) -> (-30.813, 0.4727)
  line L1101 (-30.813, 0.4727) -> (-30.4016, 0.638)
  line L1102 (-30.4016, 0.638) -> (-29.9897, 0.7853)
  line L1103 (-29.9897, 0.7853) -> (-29.5776, 0.9132)
  line L1104 (-29.5776, 0.9132) -> (-29.1656, 1.0198)
  line L1105 (-29.1656, 1.0198) -> (-28.9597, 1.0641)
  line L1106 (-28.9597, 1.0641) -> (-28.8568, 1.0838)
  line L1107 (-28.8568, 1.0838) -> (-28.754, 1.1017)
  line L1108 (-28.754, 1.1017) -> (-28.7116, 1.9099)
  circle A43 centre (0, 0) radius 0.5
  line L1109 (31.2236, 0) -> (-31.2236, 0) construction
  point P0 (15.2561, 7.5)
  point P1 (7.5, 15.2561)
  point P2 (0, 0)
  point P3 (24.6568, 7.5)
  point P4 (7.5, 24.6568)
  point P5 (0, 0)
  point P6 (-15.2561, 7.5)
  point P7 (-7.5, 15.2561)
  point P8 (-7.5, -15.2561)
  point P9 (-15.2561, -7.5)
  point P10 (15.2561, -7.5)
  point P11 (7.5, -15.2561)
  dimension "d18" = 1
  dimension "d21" = 360
  dimension "d23" = 2
  dimension "d24" = 2
  dimension "d25" = 2
  dimension "d26" = 2
  dimension "d27" = 2
  dimension "d30" = 360
  constraints: 99 point on circle, 50 end point, 42 centre point, 11 point on line, 8 tangent, 6 coincident, 5 equal radius, 4 collinear, 3 vertical, 2 parallel, 177 other
  measures "d23" radial gap between concentric circles of A1 A19
  measures "d24" distance between parallel lines of L21 L20
  measures "d25" distance between parallel lines of L22 L1
  measures "d26" radial gap between concentric circles of A3 A20
  measures "d27" radius of A21
extrude "Extrusion9" add sketch "Sketch7" along normal mid plane 1 contours L2 A1 L7 A0 | A3 L20 A1 L1 | L8 A1 L9 A3 | A3 L18 A1 L19 | L10 A1 L11 A3 | A3 L16 A1 L17 | L12 A1 L13 A3 | A3 L14 A1 L15
extrude "Extrusion11" add sketch "Sketch7" along normal mid plane 5 contours A2 L1 A1 L2 | L7 A1 L8 A4 | A3 L19 A1 L20 | L9 A1 L10 A3 | A3 L17 A1 L18 | L11 A1 L12 A3 | A3 L15 A1 L16 | L13 A1 L14 A3
extrude "Extrusion12" add sketch "Sketch7" along normal mid plane 5 contours L29 L30 L31 L32 L33 L34 L35 L36 L37 L38 L39 L40 L41 L42 L43 L44 L45 L46 L47 L48 L49 L50 L51 L52 L53 L54 L55 L56 L57 L58 L59 L60 L61 L62 L63 L64 L65 L66 L67 L68 L69 L70 L71 L72 L73 L74 L75 L76 L77 L78 L79 L80 L81 L82 L83 L84 L85 L86 L87 L88 L89 L90 L91 L92 L93 L94 L95 L96 L97 L98 L99 L100 L101 L102 L103 L104 L105 L106 L107 L108 L109 L110 L111 L112 L113 L114 L115 L116 L117 L118 L119 L120 L121 L122 L123 L124 L125 L126 L127 L128 L129 L130 L131 L132 L133 L134 L135 L136 L137 L138 L139 L140 L141 L142 L143 L144 L145 L146 L147 L148 L149 L150 L151 L152 L153 L154 L155 L156 L157 L158 L159 L160 L161 L162 L163 L164 L165 L166 L167 L168 L169 L170 L171 L172 L173 L174 L175 L176 L177 L178 L179 L180 L181 L182 L183 L184 L185 L186 L187 L188 L189 L190 L191 L192 L193 L194 L195 L196 L197 L198 L199 L200 L201 L202 L203 L204 L205 L206 L207 L208 L209 L210 L211 L212 L213 L214 L215 L216 L217 L218 L219 L220 L221 L222 L223 L224 L225 L226 L227 L228 L229 L230 L231 L232 L233 L234 L235 L236 L237 L238 L239 L240 L241 L242 L243 L244 L245 L246 L247 L248 L249 L250 L251 L252 L253 L254 L255 L256 L257 L258 L259 L260 L261 L262 L263 L264 L265 L266 L267 L268 L269 L270 L271 L272 L273 L274 L275 L276 L277 L278 L279 L280 L281 L282 L283 L284 L285 L286 L287 L288 L289 L290 L291 L292 L293 L294 L295 L296 L297 L298 L299 L300 L301 L302 L303 L304 L305 L306 L307 L308 L309 L310 L311 L312 L313 L314 L315 L316 L317 L318 L319 L320 L321 L322 L323 L324 L325 L326 L327 L328 L329 L330 L331 L332 L333 L334 L335 L336 L337 L338 L339 L340 L341 L342 L343 L344 L345 L346 L347 L348 L349 L350 L351 L352 L353 L354 L355 L356 L357 L358 L359 L360 L361 L362 L363 L364 L365 L366 L367 L368 L369 L370 L371 L372 L373 L374 L375 L376 L377 L378 L379 L380 L381 L382 L383 L384 L385 L386 L387 L388 L389 L390 L391 L392 L393 L394 L395 L396 L397 L398 L399 L400 L401 L402 L403 L404 L405 L406 L407 L408 L409 L410 L411 L412 L413 L414 L415 L416 L417 L418 L419 L420 L421 L422 L423 L424 L425 L426 L427 L428 L429 L430 L431 L432 L433 L434 L435 L436 L437 L438 L439 L440 L441 L442 L443 L444 L445 L446 L447 L448 L449 L450 L451 L452 L453 L454 L455 L456 L457 L458 L459 L460 L461 L462 L463 L464 L465 L466 L467 L468 L469 L470 L471 L472 L473 L474 L475 L476 L477 L478 L479 L480 L481 L482 L483 L484 L485 L486 L487 L488 L489 L490 L491 L492 L493 L494 L495 L496 L497 L498 L499 L500 L501 L502 L503 L504 L505 L506 L507 L508 L509 L510 L511 L512 L513 L514 L515 L516 L517 L518 L519 L520 L521 L522 L523 L524 L525 L526 L527 L528 L529 L530 L531 L532 L533 L534 L535 L536 L537 L538 L539 L540 L541 L542 L543 L544 L545 L546 L547 L548 L549 L550 L551 L552 L553 L554 L555 L556 L557 L558 L559 L560 L561 L562 L563 L564 L565 L566 L567 L568 L569 L570 L571 L572 L573 L574 L575 L576 L577 L578 L579 L580 L581 L582 L583 L584 L585 L586 L587 L588 L589 L590 L591 L592 L593 L594 L595 L596 L597 L598 L599 L600 L601 L602 L603 L604 L605 L606 L607 L608 L609 L610 L611 L612 L613 L614 L615 L616 L617 L618 L619 L620 L621 L622 L623 L624 L625 L626 L627 L628 L629 L630 L631 L632 L633 L634 L635 L636 L637 L638 L639 L640 L641 L642 L643 L644 L645 L646 L647 L648 L649 L650 L651 L652 L653 L654 L655 L656 L657 L658 L659 L660 L661 L662 L663 L664 L665 L666 L667 L668 L669 L670 L671 L672 L673 L674 L675 L676 L677 L678 L679 L680 L681 L682 L683 L684 L685 L686 L687 L688 L689 L690 L691 L692 L693 L694 L695 L696 L697 L698 L699 L700 L701 L702 L703 L704 L705 L706 L707 L708 L709 L710 L711 L712 L713 L714 L715 L716 L717 L718 L719 L720 L721 L722 L723 L724 L725 L726 L727 L728 L729 L730 L731 L732 L733 L734 L735 L736 L737 L738 L739 L740 L741 L742 L743 L744 L745 L746 L747 L748 L749 L750 L751 L752 L753 L754 L755 L756 L757 L758 L759 L760 L761 L762 L763 L764 L765 L766 L767 L768 L769 L770 L771 L772 L773 L774 L775 L776 L777 L778 L779 L780 L781 L782 L783 L784 L785 L786 L787 L788 L789 L790 L791 L792 L793 L794 L795 L796 L797 L798 L799 L800 L801 L802 L803 L804 L805 L806 L807 L808 L809 L810 L811 L812 L813 L814 L815 L816 L817 L818 L819 L820 L821 L822 L823 L824 L825 L826 L827 L828 L829 L830 L831 L832 L833 L834 L835 L836 L837 L838 L839 L840 L841 L842 L843 L844 L845 L846 L847 L848 L849 L850 L851 L852 L853 L854 L855 L856 L857 L858 L859 L860 L861 L862 L863 L864 L865 L866 L867 L868 L869 L870 L871 L872 L873 L874 L875 L876 L877 L878 L879 L880 L881 L882 L883 L884 L885 L886 L887 L888 L889 L890 L891 L892 L893 L894 L895 L896 L897 L898 L899 L900 L901 L902 L903 L904 L905 L906 L907 L908 L909 L910 L911 L912 L913 L914 L915 L916 L917 L918 L919 L920 L921 L922 L923 L924 L925 L926 L927 L928 L929 L930 L931 L932 L933 L934 L935 L936 L937 L938 L939 L940 L941 L942 L943 L944 L945 L946 L947 L948 L949 L950 L951 L952 L953 L954 L955 L956 L957 L958 L959 L960 L961 L962 L963 L964 L965 L966 L967 L968 L969 L970 L971 L972 L973 L974 L975 L976 L977 L978 L979 L980 L981 L982 L983 L984 L985 L986 L987 L988 L989 L990 L991 L992 L993 L994 L995 L996 L997 L998 L999 L1000 L1001 L1002 L1003 L1004 L1005 L1006 L1007 L1008 L1009 L1010 L1011 L1012 L1013 L1014 L1015 L1016 L1017 L1018 L1019 L1020 L1021 L1022 L1023 L1024 L1025 L1026 L1027 L1028 L1029 L1030 L1031 L1032 L1033 L1034 L1035 L1036 L1037 L1038 L1039 L1040 L1041 L1042 L1043 L1044 L1045 L1046 L1047 L1048 L1049 L1050 L1051 L1052 L1053 L1054 L1055 L1056 L1057 L1058 L1059 L1060 L1061 L1062 L1063 L1064 L1065 L1066 L1067 L1068 L1069 L1070 L1071 L1072 L1073 L1074 L1075 L1076 L1077 L1078 L1079 L1080 L1081 L1082 L1083 L1084 L1085 L1086 L1087 L1088 L1089 L1090 L1091 L1092 L1093 L1094 L1095 L1096 L1097 L1098 L1099 L1100 L1101 L1102 L1103 L1104 L1105 L1106 L1107 L1108
equation "\"d18\" = Gear_tooth_wall_thickness"
equation "\"d23\" = Gear60_lightener_hole_offset"
equation "\"d24\" = d23"
equation "\"d25\" = d23"
equation "\"d26\" = d25"
equation "\"d27\" = Gear60_lightener_hole_fillet"
equation "\"d32\" = Inner_thickness"
equation "\"Gear60_lightener_hole_offset\" = 2"
equation "\"Gear60_lightener_hole_fillet\" = 2"
equation "\"Gear_tooth_wall_thickness\" = 1"
equation "\"Inner_thickness\" = 1"
body "Solid4"
